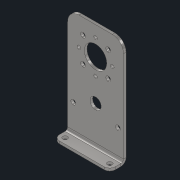
# Autodesk Inventor part: plate8
Saved by Autodesk Inventor 2021 (Build 250183000, 183)
## iProperties
Created: 2021-07-30
Part Number: plate8
Material: 鋼、炭素鋼
Document SubType Name: Sheet Metal
Designer: yuta0
Density: 7.85 g/cm^3
Sheet Metal Rule: Default_mm
Appearance: 半つや出し
購入先: Meviy
在庫数: 0.0
Author: yuta0
Autodesk Inventor part; units mm, degrees
ref_plane "YZ Plane" through (0, 0, 0) normal (1, 0, 0) x (0, 1, 0)
ref_plane "XZ Plane" through (0, 0, 0) normal (0, 1, 0) x (-1, 0, 0)
ref_plane "XY Plane" through (0, 0, 0) normal (0, 0, 1) x (1, 0, 0)
sketch "スケッチ1" plane through (0, 0, 0) normal (0, 0, 1) x (1, 0, 0)
  line L0 (-25, -71.3) -> (25, -71.3)
  line L1 (25, -71.3) -> (25, 25)
  line L2 (25, 25) -> (-25, 25)
  line L3 (-25, 25) -> (-25, -71.3)
  line L4 (-25, -71.3) -> (25, 25) construction
  line L5 (25, -71.3) -> (-25, 25) construction
  circle A0 centre (0, 0) radius 19 construction
  point P0 (0, -23.15)
  point P1 (0, -23.15)
  dimension "d0" = 38
  dimension "d1" = 50
  dimension "d2" = 25
  dimension "d3" = 71.3
  measures "d0" diameter of A0
  measures "d1" distance of L1.end L2.end
  measures "d2" distance from line of L2 point (0, 0)
  measures "d3" distance from line of L0 point (0, 0)
extrude "プレート1" add sketch "スケッチ1" along normal blind 2.3
sketch "スケッチ9" plane through (25, -69, 0) normal (0, -1, 0) x (1, 0, 0)
  line L0 (-50, 0) -> (0, 0)
  line L1 (0, 0) -> (0, 14.6)
  line L2 (0, 14.6) -> (-50, 14.6)
  line L3 (-50, 14.6) -> (-50, 0)
  constraints: 6 end point, 1 horizontal, 1 perpendicular, 1 vertical
edge flange "フランジ3" height 14.6 angle 90 thickness 2.3 bend radius 2.3 thickness toward (0, -1, 0) relief straight relief width 2.3 relief depth 1.15 edges at (0, -71.3, 2.3) wall of the first edge with corners at (-25, -69, 0) (25, -69, 0) (25, -69, 14.6) (-25, -69, 14.6)
bend "曲げ3"
corner "コーナー3"
fillet "コーナーR1" radius 5 2 edges at (-25, -70.15, 14.6) (25, -70.15, 14.6)
sketch "スケッチ4" plane through (0, 0, 2.3) normal (0, 0, 1) x (1, 0, 0)
  circle A0 centre (0, 0) radius 15
  point P0 (0, 15)
  point P1 (-15, 0)
  point P2 (0, -15)
  point P3 (15, 0)
  dimension "d26" = 30
  dimension "d29" = 360
  constraints: 1 coincident, 1 vertical alignment, 7 other
hole "穴1" at (0, 15, 2.3) at (-15, 0, 2.3) at (0, -15, 2.3) at (15, 0, 2.3) direction (0, 0, -1) diameter 3.2 end through all clearance for "Flat Head Machine Screw" size "M3" standard "Ansi Metric M Profile"
sketch "スケッチ5" plane through (0, 0, 2.3) normal (0, 0, 1) x (1, 0, 0)
  circle A0 centre (0, 0) radius 16
  point P0 (-11.3137, 11.3137)
  point P1 (-11.3137, -11.3137)
  point P2 (11.3137, -11.3137)
  point P3 (11.3137, 11.3137)
  dimension "d38" = 32
  dimension "d41" = 360
  constraints: 1 coincident, 1 horizontal alignment, 8 other
hole "穴2" at (-11.3137, 11.3137, 2.3) at (-11.3137, -11.3137, 2.3) at (11.3137, -11.3137, 2.3) at (11.3137, 11.3137, 2.3) direction (0, 0, -1) diameter 4.3 end through all clearance for "Flat Head Machine Screw" size "M4" standard "Ansi Metric M Profile"
sketch "スケッチ6" plane through (0, 0, 2.3) normal (0, 0, 1) x (1, 0, 0)
  circle A0 centre (0, 0) radius 10
  dimension "d50" = 20
  constraints: 1 centre point, 1 coincident
  measures "d50" diameter of A0
extrude "押し出し1" cut sketch "スケッチ6" against normal blind 10
sketch "スケッチ7" plane through (-25, -69, -2.3) normal (0, 1, 0) x (1, 0, 0)
  line L0 (5, -16.9) -> (45, -16.9) projected
  line L1 (0, -6.9) -> (0, -11.9) projected
  line L2 (50, -6.9) -> (50, -11.9) projected
  point P0 (18, -2.3)
  point P1 (45, -11.9)
  point P2 (5, -11.9)
  dimension "d76" = 5
  dimension "d77" = 5
  dimension "d78" = 5
  constraints: 1 horizontal alignment
  measures "d76" distance from line of L0 point (5, -11.9)
  measures "d77" distance from line of L1 point (5, -11.9)
  measures "d78" distance from line of L2 point (45, -11.9)
hole "穴3" at (20, -69, 9.6) at (-20, -69, 9.6) direction (0, -1, 0) diameter 4.3 end through all clearance for "Flat Head Machine Screw" size "M4" standard "Ansi Metric M Profile"
fillet "コーナーR3" radius 10 2 edges at (-25, 25, 1.15) (25, 25, 1.15)
sketch "スケッチ10" plane through (0, 0, 0) normal (0, 0, -1) x (-1, 0, 0)
  line L0 (-25, -66.7) -> (-25, 15) projected
  line L1 (25, 15) -> (25, -66.7) projected
  circle A0 centre (-20, -44.5) radius 4
  circle A1 centre (0, 0) radius 45
  point P0 (20, -44.5)
  dimension "d80" = 5
  dimension "d81" = 5
  dimension "d82" = 44.5
  dimension "d83" = 8
  dimension "d84" = 90
  constraints: 2 centre point, 2 coincident, 1 horizontal alignment
  measures "d80" distance from line of L0 point (-20, -44.5)
  measures "d81" distance from line of L1 point (20, -44.5)
  measures "d82" vertical distance of point (0, 0) point (-20, -44.5)
  measures "d83" diameter of A0
  measures "d84" diameter of A1
hole "穴4" at (20, -44.5, 0) at (-20, -44.5, 0) direction (0, 0, 1) diameter 4.3 end through all clearance for "Flat Head Machine Screw" size "M4" standard "Ansi Metric M Profile"
sketch "スケッチ11" plane through (0, 0, 2.3) normal (0, 0, 1) x (1, 0, 0)
  circle A0 centre (0, -36) radius 5
  point P0 (0, 0)
  dimension "d92" = 10
  dimension "d93" = 36
  constraints: 1 centre point, 1 vertical alignment
  measures "d92" diameter of A0
  measures "d93" distance of point (0, 0) A0.centre
extrude "押し出し3" cut sketch "スケッチ11" against normal blind 10
equation "\"d36\" = Thickness"
equation "\"d48\" = Thickness"
equation "\"d77\" = d76"
equation "\"d61\" = Thickness"
equation "\"d90\" = Thickness"
equation "\"d4\" = Thickness"
equation "\"d66\" = BendReliefWidth"
equation "\"d67\" = BendReliefDepth"
equation "\"d68\" = MinimumRemnant"
equation "\"d69\" = TransitionRadius"
equation "\"d72\" = BendRadius"
equation "\"d73\" = CornerReliefSize"
equation "\"d74\" = GapSize"
equation "\"d75\" = JacobiRadiusSize"
equation "\"d2\" = 0.5 * d1"
equation "\"BendRadius\" = Thickness"
equation "\"BendReliefWidth\" = Thickness"
equation "\"BendReliefDepth\" = 0.5 * Thickness"
equation "\"CornerReliefSize\" = 4 * Thickness"
equation "\"MinimumRemnant\" = 2 * Thickness"
equation "\"TransitionRadius\" = BendRadius"
equation "\"JacobiRadiusSize\" = BendRadius"
equation "\"GapSize\" = Thickness"
equation "\"Thickness\" = 2.3"
